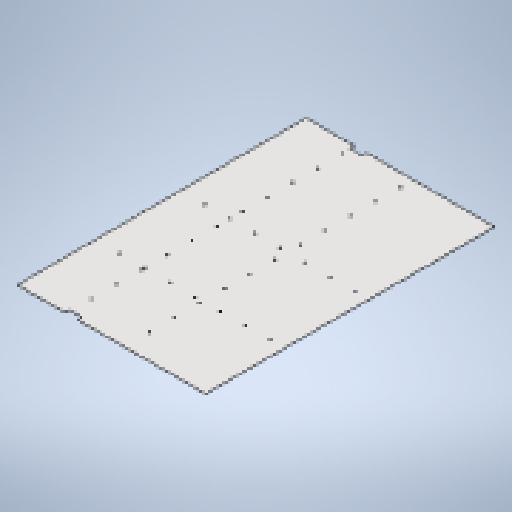
# Autodesk Inventor part: GnG frame 2 floor sheet 8
Saved by Autodesk Inventor 2025 (Build 290162010, 162A)
## iProperties
Created: 2025-10-28
Part Number: GnG frame 2 floor sheet 8
Material: Stainless Steel
Document SubType Name: Sheet Metal
Designer: admin
Mass: 280.619 g
Surface Area: 364.406 cm^2
Volume: 35.0774 cm^3
Density: 8 g/cm^3
Sheet Metal Rule: AISI304 3mm Die 32
Sheet Metal Width: 1500,000 mm
Sheet Metal Length: 2300,000 mm
Sheet Metal Area: 3450000,000 mm^2
Appearance: Default
Flat Pattern Width: 150 cm
Flat Pattern Length: 230 cm
Flat Pattern Area: 34500 cm^2
Author: admin
Autodesk Inventor part; units mm, degrees
ref_plane "YZ Plane" through (0, 0, 0) normal (1, 0, 0) x (0, 1, 0)
ref_plane "XZ Plane" through (0, 0, 0) normal (0, 1, 0) x (-1, 0, 0)
ref_plane "XY Plane" through (0, 0, 0) normal (0, 0, 1) x (1, 0, 0)
sketch "Sketch1" plane through (0, 0, 0) normal (0, 0, 1) x (1, 0, 0)
  line L0 (0, 0) -> (-1500, 0)
  line L1 (-1500, 0) -> (-1500, -2300)
  line L2 (-1500, -2300) -> (0, -2300)
  line L3 (0, -2300) -> (0, 0)
  line L4 (0, 0) -> (-65, 0)
  line L5 (-65, 0) -> (-65, -35)
  line L6 (-65, -35) -> (0, -35)
  line L7 (0, -35) -> (0, 0)
  line L8 (0, -2300) -> (-65, -2300)
  line L9 (-65, -2300) -> (-65, -2265)
  line L10 (-65, -2265) -> (0, -2265)
  line L11 (0, -2265) -> (0, -2300)
  line L12 (-1500, 0) -> (-1435, 0)
  line L13 (-1435, 0) -> (-1435, -35)
  line L14 (-1435, -35) -> (-1500, -35)
  line L15 (-1500, -35) -> (-1500, 0)
  line L16 (-1500, -2300) -> (-1435, -2300)
  line L17 (-1435, -2300) -> (-1435, -2265)
  line L18 (-1435, -2265) -> (-1500, -2265)
  line L19 (-1500, -2265) -> (-1500, -2300)
  line L20 (-1120, -2300) -> (-1020, -2300)
  line L21 (-1020, -2300) -> (-1020, -2265)
  line L22 (-1020, -2265) -> (-1120, -2265)
  line L23 (-1120, -2265) -> (-1120, -2300)
  line L24 (-1120, 0) -> (-1020, 0)
  line L25 (-1020, 0) -> (-1020, -35)
  line L26 (-1020, -35) -> (-1120, -35)
  line L27 (-1120, -35) -> (-1120, 0)
  point P0 (0, -35)
  point P1 (-65, 0)
  point P2 (0, -2265)
  point P3 (-1020, -2300)
  point P4 (-1020, 0)
  point P5 (-1435, 0)
  dimension "d22" = 1500
  dimension "d23" = 2300
  dimension "d24" = 65
  dimension "d25" = 35
  dimension "d28" = 100
  dimension "d29" = 955
  measures "d22" distance of L2.end L1.end
  measures "d23" distance of L1.end L0.end
  measures "d24" distance of L6.end L5.end
  measures "d25" distance of L5.end L4.end
  measures "d28" distance of L25.end L26.end
  measures "d29" distance between parallel lines of L5 L25
extrude "Plate1" add sketch "Sketch1" along normal blind 3 contours L3 L6 L5 L0 | L5 L6 L3 L10 L9 L2 L21 L22 L23 L17 L18 L1 L14 L13 L0 L27 L26 L25 | L3 L2 L9 L10 | L13 L14 L1 L0 | L18 L17 L2 L1
sketch "Sketch5" plane through (0, 0, 3) normal (0, 0, 1) x (1, 0, 0)
  line L0 (0, 0) -> (-100, 0) construction
  line L1 (0, -2) -> (0, 0) construction
  line L2 (-112, 0) -> (-107.0911, 0) construction
  line L3 (-107.0911, 0) -> (-112.0911, 0)
  line L4 (-112.0911, 0) -> (-112.0911, -2)
  line L5 (-112.0911, -2) -> (-107.0911, -2)
  line L6 (-107.0911, -2) -> (-107.0911, 0)
  line L7 (-112.0911, 0) -> (-116.7331, 0) construction
  line L8 (-116.7331, 0) -> (-121.7331, 0)
  line L9 (-121.7331, 0) -> (-121.7331, -2)
  line L10 (-121.7331, -2) -> (-116.7331, -2)
  line L11 (-116.7331, -2) -> (-116.7331, 0)
  circle A0 centre (-126.7401, 0) radius 2.5
  circle A1 centre (-133.5151, 0) radius 2.5
  point P0 (0, 0)
  dimension "d36" = 2
  dimension "d37" = 2
  dimension "d38" = 5
  dimension "d64" = 5
  constraints: 24 end point, 5 horizontal, 4 parallel, 2 centre point, 2 coincident, 2 perpendicular, 1 collinear, 1 equal radius
  measures "d36" distance of L4.end L4.start
  measures "d37" distance of L9.end L9.start
  measures "d38" diameter of A0
  measures "d64" distance of L9.end L11.start
extrude "Cut1" cut sketch "Sketch5" against normal blind 3
sketch "Sketch6" plane through (0, 0, 3) normal (0, 0, 1) x (1, 0, 0)
  line L0 (-107.0911, 0) -> (0, 0) construction
  arc A0 (-129.2401, 0) -> (-124.2401, 0) centre (-126.7401, 0) ccw construction
  line L1 (-131.0151, 0) -> (-129.2401, 0) construction
  arc A1 (-136.0151, 0) -> (-131.0151, 0) centre (-133.5151, 0) ccw construction
  line L2 (-1020, 0) -> (-136.0151, 0) construction
  line L3 (-1020, -35) -> (-1020, 0) construction
  line L4 (-1120, -35) -> (-1020, -35) construction
  line L5 (-1120, 0) -> (-1120, -35) construction
  line L6 (-1500, 0) -> (-1120, 0) construction
  line L7 (-1500, -2300) -> (-1500, 0) construction
  line L8 (-1120, -2300) -> (-1500, -2300) construction
  line L9 (-1120, -2265) -> (-1120, -2300) construction
  line L10 (-1020, -2265) -> (-1120, -2265) construction
  line L11 (-1020, -2300) -> (-1020, -2265) construction
  line L12 (0, -2300) -> (-1020, -2300) construction
  line L13 (0, 0) -> (0, -2300) construction
  line L14 (0, -2300) -> (0, 0) construction
  line L15 (0, -1000) -> (-1500, -1000) construction
  line L16 (-1500, -1675) -> (0, -1675) construction
  line L17 (-650, 0) -> (-650, -2300) construction
  line L18 (-1110, -2300) -> (-1110, 0) construction
  circle A2 centre (-650, -2100) radius 7.5
  circle A3 centre (-1110, -2100) radius 7.5
  circle A4 centre (-1310, -1675) radius 7.5
  circle A5 centre (-1310, -1000) radius 7.5
  circle A6 centre (-650, -1900) radius 7.5
  circle A7 centre (-1110, -1900) radius 7.5
  circle A8 centre (-650, -1700) radius 7.5
  circle A9 centre (-1110, -1700) radius 7.5
  circle A10 centre (-650, -1500) radius 7.5
  circle A11 centre (-1110, -1500) radius 7.5
  circle A12 centre (-650, -1300) radius 7.5
  circle A13 centre (-1110, -1300) radius 7.5
  circle A14 centre (-650, -1100) radius 7.5
  circle A15 centre (-1110, -1100) radius 7.5
  circle A16 centre (-650, -900) radius 7.5
  circle A17 centre (-1110, -900) radius 7.5
  circle A18 centre (-650, -700) radius 7.5
  circle A19 centre (-1110, -700) radius 7.5
  circle A20 centre (-650, -500) radius 7.5
  circle A21 centre (-1110, -500) radius 7.5
  circle A22 centre (-650, -300) radius 7.5
  circle A23 centre (-1110, -300) radius 7.5
  circle A24 centre (-650, -100) radius 7.5
  circle A25 centre (-1110, -100) radius 7.5
  circle A26 centre (-1110, -1675) radius 7.5
  circle A27 centre (-1110, -1000) radius 7.5
  circle A28 centre (-910, -1675) radius 7.5
  circle A29 centre (-910, -1000) radius 7.5
  circle A30 centre (-710, -1675) radius 7.5
  circle A31 centre (-710, -1000) radius 7.5
  circle A32 centre (-510, -1675) radius 7.5
  circle A33 centre (-510, -1000) radius 7.5
  circle A34 centre (-310, -1675) radius 7.5
  circle A35 centre (-310, -1000) radius 7.5
  circle A36 centre (-110, -1675) radius 7.5
  circle A37 centre (-110, -1000) radius 7.5
  line L19 (-107.0911, 0) -> (-107.0911, -2) projected
  line L20 (-107.0911, -2) -> (-112.0911, -2) projected
  line L21 (-112.0911, -2) -> (-112.0911, 0) projected
  line L22 (-116.7331, 0) -> (-112.0911, 0) projected
  line L23 (-116.7331, 0) -> (-116.7331, -2) projected
  line L24 (-116.7331, -2) -> (-121.7331, -2) projected
  line L25 (-121.7331, -2) -> (-121.7331, 0) projected
  line L26 (-124.2401, 0) -> (-121.7331, 0) projected
  dimension "d41" = 390
  dimension "d42" = 850
  dimension "d43" = 1300
  dimension "d44" = 625
  dimension "d45" = 15
  dimension "d46" = 200
  dimension "d47" = 190
  dimension "d50" = 200
  dimension "d57" = 200
  constraints: 36 centre point, 12 point on line, 8 end point, 4 perpendicular, 3 equal radius, 1 horizontal, 1 horizontal alignment, 1 vertical, 1 vertical alignment, 64 other
  measures "d41" distance between parallel lines of L7 L18
  measures "d42" distance between parallel lines of L7 L17
  measures "d43" distance between parallel lines of L8 L15
  measures "d44" distance between parallel lines of L8 L16
  measures "d45" diameter of A2
  measures "d46" distance from line of L8 A2.centre
  measures "d47" distance from line of L7 A5.centre
  measures "d50" distance of A2.centre A6.centre
  measures "d57" distance of A4.centre A26.centre
extrude "Cut2" cut sketch "Sketch6" against normal blind 3
equation "\"d39\" = Thickness"
equation "\"d50\" = d46"
equation "\"d57\" = d46"
equation "\"d62\" = Thickness"
equation "\"d2\" = Thickness"
equation "\"BendReliefWidth\" = Thickness"
equation "\"BendReliefDepth\" = 0.5 * Thickness"
equation "\"CornerReliefSize\" = 4 * Thickness"
equation "\"MinimumRemnant\" = 2 * Thickness"
equation "\"TransitionRadius\" = BendRadius"
equation "\"JacobiRadiusSize\" = BendRadius"
equation "\"GapSize\" = Thickness"
equation "\"Thickness\" = 3"
equation "\"BendRadius\" = 5"
body "Solid1"
